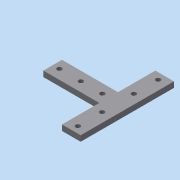
# Autodesk Inventor part: side corner brackets
Saved by Autodesk Inventor 2015 (Build 190159000, 159)
## iProperties
Created: 2016-09-09
Part Number: side corner brackets
Material: Generic
Document SubType Name: Modeling
Designer: Dustin
Density: 1 g/cm^3
Appearance: Default
Author: Dustin
Autodesk Inventor part; units mm, degrees
ref_plane "YZ Plane" through (0, 0, 0) normal (1, 0, 0) x (0, 1, 0)
ref_plane "XZ Plane" through (0, 0, 0) normal (0, 1, 0) x (-1, 0, 0)
ref_plane "XY Plane" through (0, 0, 0) normal (0, 0, 1) x (1, 0, 0)
sketch "Sketch1" plane through (0, 0, 0) normal (0, 0, 1) x (1, 0, 0)
  line L0 (0, 0) -> (0, 100)
  line L1 (0, 100) -> (-20, 100)
  line L2 (-20, 100) -> (-20, 60)
  line L3 (-20, 60) -> (-80, 60)
  line L4 (-80, 60) -> (-80, 40)
  line L5 (-80, 40) -> (-20, 40)
  line L6 (-20, 40) -> (-20, 0)
  line L7 (-20, 0) -> (0, 0)
  dimension "d0" = 20
  dimension "d1" = 100
  dimension "d2" = 20
  dimension "d3" = 40
  dimension "d4" = 60
  constraints: 16 end point, 6 perpendicular, 2 point on line, 1 vertical
  measures "d0" distance of L6.end L0.start
  measures "d1" distance of L0.start L0.end
  measures "d2" distance of L3.end L4.end
  measures "d3" distance of L1.end L2.end
  measures "d4" distance of L4.end L5.end
extrude "Extrusion1" add sketch "Sketch1" along normal blind 6
sketch "Sketch2" plane through (0, 0, 6) normal (0, 0, 1) x (1, 0, 0)
  line L0 (0, 100) -> (-20, 100) projected
  line L1 (-20, 60) -> (-80, 60) projected
  line L2 (-80, 40) -> (-20, 40) projected
  line L3 (-20, 0) -> (0, 0) projected
  line L4 (-20, 40) -> (-20, 0) projected
  line L5 (-20, 100) -> (-20, 60) projected
  line L6 (-80, 60) -> (-80, 40) projected
  point P0 (-10, 93)
  point P1 (-10, 67)
  point P2 (-10, 33)
  point P3 (-10, 7)
  point P4 (-73, 50.2147)
  point P5 (-50, 50.2147)
  point P6 (-27, 50.2147)
  dimension "d7" = 7
  dimension "d8" = 7
  dimension "d9" = 7
  dimension "d10" = 7
  dimension "d11" = 10
  dimension "d12" = 10
  dimension "d13" = 10
  dimension "d14" = 10
  dimension "d15" = 7
  dimension "d16" = 7
  dimension "d17" = 23
  measures "d7" distance from line of L0 point (-10, 93)
  measures "d8" distance from line of L1 point (-10, 67)
  measures "d9" distance from line of L2 point (-10, 33)
  measures "d10" distance from line of L3 point (-10, 7)
  measures "d11" distance from line of L4 point (-10, 7)
  measures "d12" distance from line of L4 point (-10, 33)
  measures "d13" distance from line of L5 point (-10, 67)
  measures "d14" distance from line of L5 point (-10, 93)
  measures "d15" distance from line of L4 point (-27, 50.215)
  measures "d16" distance from line of L6 point (-73, 50.215)
  measures "d17" distance of point (-50, 50.215) point (-73, 50.215)
hole "Hole1" at (-10, 93, 6) at (-10, 67, 6) at (-10, 33, 6) at (-10, 7, 6) at (-73, 50.2147, 6) at (-50, 50.2147, 6) at (-27, 50.2147, 6) direction (0, 0, -1) diameter 5 depth 8 tip angle 118
body "Solid1"
